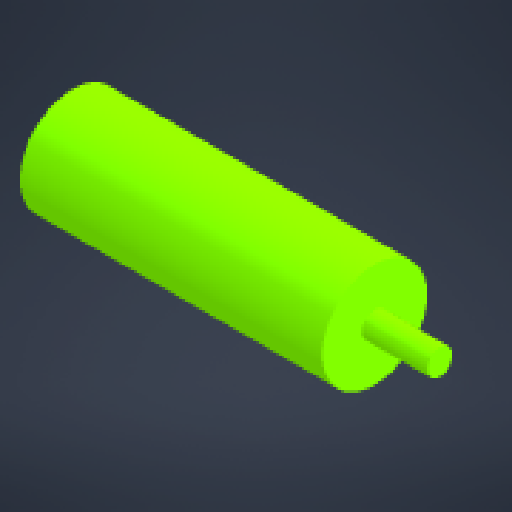
# Autodesk Inventor part: motor
Saved by Autodesk Inventor 2024 (Build 280153000, 153)
## iProperties
Created: 2023-10-10
Part Number: motor
Material: Типовые
Document SubType Name: Modeling
Designer: user
Density: 1 g/cm^3
Appearance: По умолчанию
Author: user
Autodesk Inventor part; units mm, degrees
ref_plane "YZ Plane" through (0, 0, 0) normal (1, 0, 0) x (0, 1, 0)
ref_plane "XZ Plane" through (0, 0, 0) normal (0, 1, 0) x (-1, 0, 0)
ref_plane "XY Plane" through (0, 0, 0) normal (0, 0, 1) x (1, 0, 0)
sketch "Эскиз1" plane through (0, 0, 0) normal (0, 0, 1) x (1, 0, 0)
  line L0 (0, 0) -> (0, 12.2)
  line L1 (0, 12.2) -> (30.8, 12.2)
  line L2 (33.82, 12.2) -> (70.62, 12.2)
  line L3 (70.62, 12.2) -> (70.62, 3)
  line L4 (70.62, 3) -> (85.82, 3)
  line L5 (85.82, 3) -> (85.82, 0)
  line L6 (0, 0) -> (85.82, 0)
  line L7 (30.8, 12.2) -> (32.31, 12.2)
  line L8 (32.31, 12.2) -> (33.82, 12.2)
  dimension "d0" = 3
  dimension "d1" = 85.82
  dimension "d2" = 30.8
  dimension "d3" = 36.8
  dimension "d4" = 15.2
  dimension "d5" = 12.2
  constraints: 18 end point, 4 perpendicular, 2 collinear, 2 horizontal, 2 vertical
  measures "d0" distance of L4.end L5.end
  measures "d1" horizontal distance of L4.end L0.end
  measures "d2" distance of L0.end L1.end
  measures "d3" distance of L2.start L2.end
  measures "d4" distance of L3.end L4.end
  measures "d5" distance of L0.start L0.end
revolve "Вращение1" add sketch "Эскиз1" angle 360 about axis through (0, 0, 0) along (1, 0, 0)
